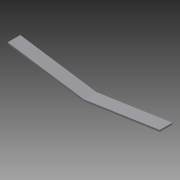
# Autodesk Inventor part: plough
Saved by Autodesk Inventor 2013 (Build 170138000, 138)
## iProperties
Created: 2013-02-04
Part Number: plough
Material: Generic
Document SubType Name: Modeling
Designer: Arpan
Density: 1 g/cm^3
Author: Arpan
Autodesk Inventor part; units mm, degrees
ref_plane "YZ Plane" through (0, 0, 0) normal (1, 0, 0) x (0, 1, 0)
ref_plane "XZ Plane" through (0, 0, 0) normal (0, 1, 0) x (-1, 0, 0)
ref_plane "XY Plane" through (0, 0, 0) normal (0, 0, 1) x (1, 0, 0)
sketch "Sketch1" plane through (0, 0, 0) normal (0, 0, 1) x (1, 0, 0)
  line L0 (0, 0) -> (0, 22.86)
  line L1 (-304.8, 0) -> (-304.8, 22.86)
  line L2 (-304.8, 22.86) -> (-152.4, 0)
  line L3 (-152.4, 0) -> (0, 22.86)
  line L4 (-304.8, 19.6495) -> (-173.8035, 0)
  line L5 (-130.9965, 0) -> (0, 19.6495)
  line L6 (-173.8035, 0) -> (-152.4, -3.2105)
  line L7 (-130.9965, 0) -> (-152.4, -3.2105)
  dimension "d0" = 22.86
  dimension "d2" = 304.8
  dimension "d4" = 3.175
  dimension "d5" = 3.175
  constraints: 16 end point, 2 collinear, 2 parallel, 2 point on line, 1 equal length, 1 vertical
  measures "d0" distance of L0.start L0.end
  measures "d2" distance of L0.start L1.start
  measures "d4" distance between parallel lines of L2 L4
  measures "d5" distance between parallel lines of L3 L5
extrude "Extrusion1" add sketch "Sketch1" along normal blind 25.4
body "Solid1"
